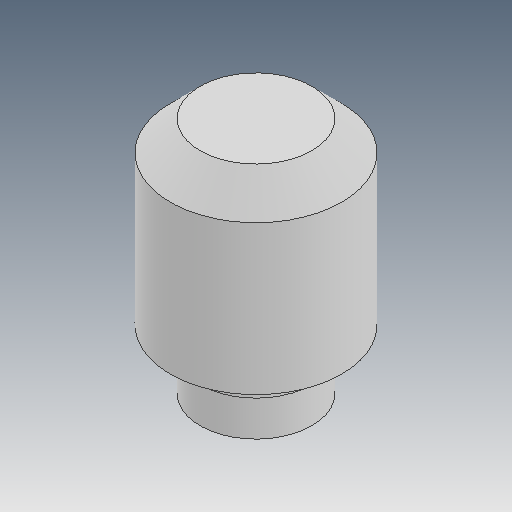
# Autodesk Inventor part: SlipersLåda 211018010
Saved by Autodesk Inventor 2020 (Build 240168000, 168)
## iProperties
Created: 2021-10-19
Part Number: SlipersLåda 211018010
Material: Generic
Document SubType Name: Modeling
Designer: dicpet001
Density: 1 g/cm^3
Appearance: Default
Author: dicpet001
Autodesk Inventor part; units mm, degrees
ref_plane "YZ Plane" through (0, 0, 0) normal (1, 0, 0) x (0, 1, 0)
ref_plane "XZ Plane" through (0, 0, 0) normal (0, 1, 0) x (-1, 0, 0)
ref_plane "XY Plane" through (0, 0, 0) normal (0, 0, 1) x (1, 0, 0)
sketch "Sketch1" plane through (0, 0, 0) normal (0, 0, 1) x (1, 0, 0)
  line L0 (0, 19.2) -> (0, -3.2) projected
  line L1 (-1.15, 0) -> (6.9, 0) projected
  line L2 (0, 0) -> (3.75, 0)
  line L3 (3.75, 0) -> (3.75, 2.382)
  line L4 (3.75, 4) -> (5.75, 4)
  line L5 (5.75, 4) -> (5.75, 14)
  line L6 (3.75, 16) -> (0, 16)
  line L7 (0, 16) -> (0, 0)
  arc A0 (3.75, 4) -> (3.4167, 3.1273) centre (3.75, 3.5) ccw
  arc A1 (3.75, 2.382) -> (3.4167, 3.1273) centre (2.75, 2.382) ccw
  line L8 (3.75, 16) -> (5.75, 14)
  point P0 (5.75, 16)
  point P1 (3.75, 3)
  dimension "d0" = 3.75
  dimension "d1" = 4
  dimension "d2" = 2
  dimension "d3" = 12
  dimension "d4" = 1
  dimension "d5" = 1
  dimension "d6" = 2
  dimension "d7" = 2
  constraints: 14 end point, 6 point on line, 5 point on circle, 3 perpendicular, 3 tangent, 2 centre point, 1 collinear, 1 vertical
  measures "d0" distance of L2.start L2.end
  measures "d1" distance of L2.end L4.start
  measures "d2" distance of L4.start L4.end
  measures "d3" distance of L4.end point (5.75, 16)
  measures "d4" diameter of A0
  measures "d5" radius of A1
  measures "d6" distance of L6.start point (5.75, 16)
  measures "d7" distance of L5.end point (5.75, 16)
revolve "Revolution1" add sketch "Sketch1" angle 360 about axis through (0, 0, 0) along (0, -1, 0)
equation "\"d7\" = d6"
body "Solid1"
